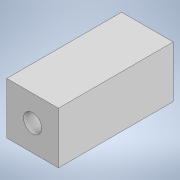
# Autodesk Inventor part: OMEGAETTE_HOUSING_V2
Saved by Autodesk Inventor 2020 (Build 240168000, 168)
## iProperties
Created: 2020-06-15
Part Number: OMEGAETTE_HOUSING_V2
Material: Generic
Document SubType Name: Modeling
Designer: Admin
Density: 1 g/cm^3
Appearance: Default
Author: Admin
Autodesk Inventor part; units mm, degrees
ref_plane "YZ Plane" through (0, 0, 0) normal (1, 0, 0) x (0, 1, 0)
ref_plane "XZ Plane" through (0, 0, 0) normal (0, 1, 0) x (-1, 0, 0)
ref_plane "XY Plane" through (0, 0, 0) normal (0, 0, 1) x (1, 0, 0)
sketch "Sketch2" plane through (0, 0, 0) normal (0, 1, 0) x (-1, 0, 0)
  line L0 (0, 0) -> (18, 0)
  line L1 (18, 0) -> (18, -40)
  line L2 (18, -40) -> (0, -40)
  line L3 (0, -40) -> (0, 0)
  dimension "d3" = 18
  dimension "d4" = 40
  constraints: 8 end point, 2 parallel, 1 horizontal, 1 perpendicular
  measures "d3" distance of L0.start L0.end
  measures "d4" distance of L0.end L1.end
extrude "Extrusion2" add sketch "Sketch2" along normal blind 5.825
sketch "Sketch3" plane through (0, 5.825, 0) normal (0, 1, 0) x (1, 0, 0)
  line L0 (-18, 0) -> (0, 0) projected
  line L1 (-18, 0) -> (-12.175, 0)
  line L2 (-12.175, 40) -> (-18, 40)
  line L3 (0, 0) -> (0, 40) projected
  line L4 (0, 0) -> (-5.825, 0)
  line L5 (-5.825, 0) -> (-5.825, 40)
  line L6 (-5.825, 40) -> (0, 40)
  line L7 (0, 40) -> (0, 0)
  line L8 (0, 40) -> (-18, 40) projected
  line L9 (-18, 0) -> (-18, 5.1947)
  line L10 (-12.175, 40) -> (-12.175, 20)
  line L11 (-12.175, 20) -> (-18, 14.175)
  line L12 (-18, 40) -> (-18, 0) projected
  line L13 (-18, 14.175) -> (-18, 40)
  line L14 (-18, 5.1947) -> (-13.3276, 9.8672)
  line L15 (-13.3276, 9.8672) -> (-13.3276, 16.8672)
  line L16 (-13.3276, 16.8672) -> (-12.175, 16.8672)
  line L17 (-12.175, 16.8672) -> (-12.175, 0)
  point P0 (0, 40)
  dimension "d8" = 5.825
  dimension "d12" = 5.825
  dimension "d13" = 6.35
  dimension "d14" = 7
  dimension "d16" = 20
  dimension "d17" = 5.825
  dimension "d18" = 45
  dimension "d19" = 16.8672
  constraints: 28 end point, 5 parallel, 4 vertical, 3 point on line, 2 horizontal, 2 perpendicular
  measures "d8" distance of L2.end L2.start
  measures "d12" distance of L5.end L6.end
  measures "d13" distance between parallel lines of L14 L11
  measures "d14" distance of L14.end L15.end
  measures "d16" distance of L2.start L10.end
  measures "d17" distance of L0.start L1.end
  measures "d18" angle of L12 L11
  measures "d19" distance between parallel lines of L1 L16
extrude "Extrusion4" add sketch "Sketch3" along normal blind 6.35 contours L9 L14 L15 L16 L17 L0 | L5 L6 L3 L0 | L12 L2 L10 L11
chamfer "Chamfer1" distance 1.152 angle 45 1 edges at (-13.3276, 9, -16.8672)
fillet "Fillet1" radius 3.175 5 edges at (-15.6638, 5.825, -7.531) (-12.175, 5.825, -8.4336) (-15.0875, 5.825, -17.0875) (-5.825, 5.825, -20) (-12.175, 5.825, -30)
sketch "Sketch4" plane through (0, 12.175, 0) normal (0, 1, 0) x (1, 0, 0)
  line L0 (0, 0) -> (0, 40) projected
  line L1 (0, 40) -> (-18, 40)
  line L2 (-18, 40) -> (-18, 0)
  line L3 (-18, 0) -> (0, 0)
  line L4 (0, 0) -> (0, 40)
  constraints: 8 end point, 2 parallel, 1 horizontal, 1 perpendicular
extrude "Extrusion5" add sketch "Sketch4" along normal blind 5.825
fillet "Fillet2" radius 3.175 5 edges at (-12.175, 12.175, -8.4336) (-5.825, 12.175, -20) (-15.0875, 12.175, -17.0875) (-15.6638, 12.175, -7.531) (-12.175, 12.175, -30)
sketch "Sketch6" plane through (0, 0, -40) normal (0, 0, -1) x (-1, 0, 0)
  circle A0 centre (9, 9) radius 7.5
  line L0 (0, 0) -> (18, 0) projected
  line L1 (0, 0) -> (0, 18) projected
  dimension "d29" = 9
  dimension "d30" = 9
  dimension "d34" = 15
  constraints: 1 centre point
  measures "d29" distance from line of L0 A0.centre
  measures "d30" distance from line of L1 A0.centre
  measures "d34" diameter of A0
extrude "Extrusion6" cut sketch "Sketch6" against normal blind 10
sketch "Sketch7" plane through (-9, 9, -30) normal (0, 0, -1) x (-1, 0, 0)
  circle A0 centre (0, 0) radius 6.25
  point P0 (-9, -9)
  dimension "d33" = 12.5
  constraints: 1 centre point
  measures "d33" diameter of A0
extrude "Extrusion7" cut sketch "Sketch7" against normal blind 9
chamfer "Chamfer2" distance 3 angle 45 6 edges at (-12.175, 9.0005, -21) (-9, 5.825, -21) (-9, 12.175, -21) (-6.7546, 11.2454, -21) (-5.825, 9.0005, -21) (-11.2454, 11.2454, -21)
chamfer "Chamfer3" distance 1.2 angle 45 1 edges at (-2.75, 9, -30)
equation "\"d17\" = d8"
body "Solid2"
